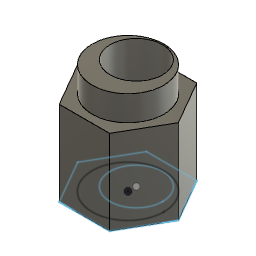
Eccentric Spacer (Autodesk Fusion 360 design; units mm, degrees)
Autodesk Fusion 360 part; units mm, degrees
sketch "Skizze1" plane through (0, 0, 0) normal (0, 1, 0) x (1, 0, 0)
  line L0 (5, 0) -> (2.5, 4.3301)
  line L1 (2.5, 4.3301) -> (-2.5, 4.3301)
  line L2 (-2.5, 4.3301) -> (-5, 0)
  line L3 (-5, 0) -> (-2.5, -4.3301)
  line L4 (-2.5, -4.3301) -> (2.5, -4.3301)
  line L5 (2.5, -4.3301) -> (5, 0)
  circle A0 centre (0, 0) radius 3.55
  circle A1 centre (0, 0.828) radius 2.6
  dimension "d1" = 10
  dimension "d2" = 7.1
  dimension "d3" = 5.2
  constraint coincident A0.centre origin
  constraint vertical A0.centre A1.centre
  measures "d1" distance of L1.end L4.end
  measures "d2" diameter of A0
  measures "d3" diameter of A1
extrude "Extrusion1" add sketch "Skizze1" along normal blind 8.4 contours L0 L1 L2 L3 L4 L5 | A0
extrude "Extrusion2" add sketch "Skizze1" along normal blind 2.5 from surface at 8.4 contours A0
named bodies: "Eccentric Spacer"
